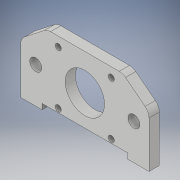
# Autodesk Inventor part: Tope riel motor
Saved by Autodesk Inventor 2019 (Build 230136000, 136)
## iProperties
Created: 2020-02-01
Part Number: Tope riel motor
Material: Generic
Document SubType Name: Modeling
Designer: Elías Sánchez
Density: 1 g/cm^3
Appearance: Default
Author: Elías Sánchez
Autodesk Inventor part; units mm, degrees
ref_plane "YZ Plane" through (0, 0, 0) normal (1, 0, 0) x (0, 1, 0)
ref_plane "XZ Plane" through (0, 0, 0) normal (0, 1, 0) x (-1, 0, 0)
ref_plane "XY Plane" through (0, 0, 0) normal (0, 0, 1) x (1, 0, 0)
sketch "Sketch1" plane through (0, 0, 0) normal (0, 0, 1) x (1, 0, 0)
  line L0 (37.5, 0) -> (37.5, 30)
  line L1 (37.5, 30) -> (22.1407, 42)
  line L2 (22.1407, 42) -> (-22.1407, 42)
  line L3 (-22.1407, 42) -> (-37.5, 30)
  line L4 (-37.5, 30) -> (-37.5, 0)
  circle A0 centre (-28.678, 21) radius 3.5
  circle A1 centre (28.678, 21) radius 3.5
  circle A2 centre (-15.5, 36.5) radius 1.75
  circle A3 centre (15.5, 36.5) radius 1.75
  circle A4 centre (-15.5, 5.5) radius 1.75
  circle A5 centre (15.5, 5.5) radius 1.75
  circle A6 centre (0, 21) radius 11.5
  line L5 (-37.5, 0) -> (-25, 0)
  line L6 (-25, 0) -> (-25, 3.2)
  line L7 (-25, 3.2) -> (25, 3.2)
  line L8 (25, 3.2) -> (25, 0)
  line L9 (25, 0) -> (37.5, 0)
  point P0 (0, 0)
  point P1 (0, 42)
  point P2 (0, 0)
  dimension "d0" = 30
  dimension "d1" = 30
  dimension "d3" = 128
  dimension "d4" = 75
  dimension "d5" = 7
  dimension "d7" = 7
  dimension "d9" = 28.678
  dimension "d10" = 28.678
  dimension "d13" = 3.5
  dimension "d14" = 3.5
  dimension "d15" = 15.5
  dimension "d16" = 15.5
  dimension "d21" = 3.5
  dimension "d22" = 3.5
  dimension "d23" = 31
  dimension "d24" = 23
  dimension "d28" = 50
  dimension "d29" = 12.5
  dimension "d30" = 3.2
  dimension "d31" = 17.8
  dimension "d32" = 2.3
  dimension "d33" = 128
  dimension "d34" = 44.2814
  dimension "d35" = 12
  dimension "d36" = 12
  dimension "d37" = 42
  constraints: 20 end point, 7 centre point, 4 horizontal alignment, 4 perpendicular, 4 vertical alignment, 2 coincident, 1 horizontal, 1 midpoint, 1 parallel, 1 point on line
  measures "d0" distance of L3.end L4.end
  measures "d1" distance of L0.start L0.end
  measures "d3" angle of L0 L1
  measures "d4" distance of L4.end L0.start
  measures "d5" diameter of A0
  measures "d7" diameter of A1
  measures "d9" horizontal distance of point (0, 0) A1.centre
  measures "d10" horizontal distance of point (0, 0) A0.centre
  measures "d13" diameter of A2
  measures "d14" diameter of A3
  measures "d15" horizontal distance of point (0, 0) A2.centre
  measures "d16" horizontal distance of point (0, 0) A3.centre
  measures "d21" diameter of A4
  measures "d22" diameter of A5
  measures "d23" distance of A5.centre A3.centre
  measures "d24" diameter of A6
  measures "d28" distance of L6.end L7.end
  measures "d29" distance of L8.end L0.start
  measures "d30" distance between parallel lines of L9 L7
  measures "d31" distance from line of L7 A6.centre
  measures "d32" distance from line of L7 A4.centre
  measures "d33" angle of L3 L4
  measures "d34" distance of L1.end L2.end
  measures "d35" vertical distance of L0.end L1.end
  measures "d36" vertical distance of L2.end L3.end
  measures "d37" distance from line of L2 point (0, 0)
extrude "Extrusion2" add sketch "Sketch1" along normal blind 6
fillet "Fillet2" radius 6 4 edges at (22.1407, 42, 3) (37.5, 30, 3) (-22.1407, 42, 3) (-37.5, 30, 3)
equation "\"d1\" = d0"
equation "\"d7\" = d5"
equation "\"d10\" = d9"
equation "\"d14\" = d13"
equation "\"d16\" = d15"
equation "\"d21\" = d13"
equation "\"d22\" = d13"
body "Solid2"
